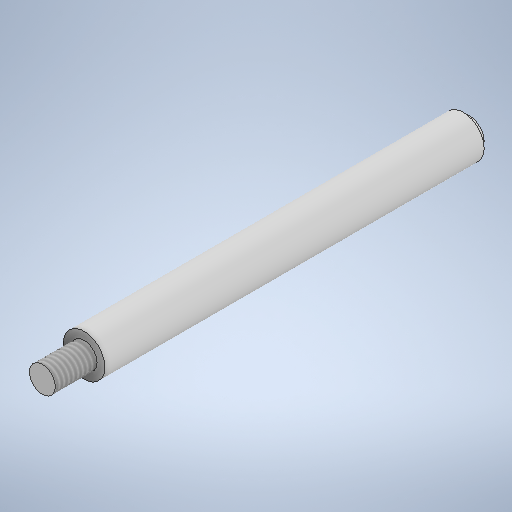
# Autodesk Inventor part: 07
Saved by Autodesk Inventor 2025.1 (Build 291241000, 241)
## iProperties
Created: 2024-09-12
Part Number: 07
Material: Generisch
Document SubType Name: Modeling
Designer: ffogue
Density: 1 g/cm^3
Appearance: Vorgabe
Author: ffogue
Autodesk Inventor part; units mm, degrees
ref_plane "YZ Plane" through (0, 0, 0) normal (1, 0, 0) x (0, 1, 0)
ref_plane "XZ Plane" through (0, 0, 0) normal (0, 1, 0) x (-1, 0, 0)
ref_plane "XY Plane" through (0, 0, 0) normal (0, 0, 1) x (1, 0, 0)
sketch "Sketch1" plane through (0, 0, 0) normal (0, 0, 1) x (1, 0, 0)
  line L0 (0, 0) -> (0, 41)
  line L1 (0, 41) -> (2, 41)
  line L2 (2, 41) -> (2, 4)
  line L3 (2, 4) -> (1.25, 4)
  line L4 (1.25, 4) -> (1.25, 0)
  line L5 (1.25, 0) -> (0, 0)
  dimension "d0" = 41
  dimension "d1" = 4
  dimension "d2" = 4
  dimension "d3" = 2.5
  constraints: 12 end point, 5 perpendicular, 1 vertical
  measures "d0" distance between parallel lines of L5 L1
  measures "d1" distance of L3.end L4.end
  measures "d2" diameter of L2 L0
  measures "d3" diameter of L4 L0
revolve "Revolution1" add sketch "Sketch1" angle 360 about axis through (0, 0, 0) along (0, 1, 0)
thread "Thread1" size "M2.5x0.45" class "6g" standard "ISO Metric profile" full length
chamfer "Chamfer1" distance 0.6 angle 45 1 edges at (-2, 41, 0)
body "Solid1"
